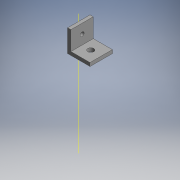
# Autodesk Inventor part: Part5
Saved by Autodesk Inventor 2016 (Build 200138000, 138)
## iProperties
Created: 2018-01-23
Part Number: Part5
Material: Generic
Document SubType Name: Modeling
Designer: student
Density: 1 g/cm^3
Appearance: Default
Author: student
Autodesk Inventor part; units mm, degrees
ref_plane "YZ Plane" through (0, 0, 0) normal (1, 0, 0) x (0, 1, 0)
ref_plane "XZ Plane" through (0, 0, 0) normal (0, 1, 0) x (-1, 0, 0)
ref_plane "XY Plane" through (0, 0, 0) normal (0, 0, 1) x (1, 0, 0)
sketch "Sketch1" plane through (0, 0, 0) normal (1, 0, 0) x (0, 1, 0)
  circle A0 centre (77.4226, -114.2734) radius 1.75 projected
  line L0 (66.4726, -104.7484) -> (66.4726, -123.7984) projected
  line L1 (66.4726, -104.7484) -> (85.5226, -104.7484) projected
  line L2 (85.5226, -123.7984) -> (85.5226, -104.7484) projected
  line L3 (66.4726, -123.7984) -> (85.5226, -123.7984) projected
  point P0 (0, 0)
extrude "Extrusion1" add sketch "Sketch1" along normal blind 2.794
sketch "Sketch3" plane through (2.794, 0, 0) normal (1, 0, 0) x (0, 0, -1)
  line L0 (104.7484, 66.4726) -> (123.7984, 66.4726) projected
  line L1 (104.7484, 85.5226) -> (104.7484, 66.4726) projected
  line L2 (104.7484, 66.4726) -> (104.7484, 69.3936)
  line L3 (104.7484, 66.4726) -> (107.6694, 66.4726) construction
  line L4 (123.7984, 66.4726) -> (123.7984, 85.5226) projected
  line L5 (123.7984, 66.4726) -> (123.7984, 69.3936)
  line L6 (123.7984, 66.4726) -> (126.7194, 66.4726) construction
  line L7 (123.7984, 69.3936) -> (104.7484, 69.3936)
  point P0 (0, 0)
  dimension "d2" = 2.921
  dimension "d3" = 90
  dimension "d4" = 2.921
  dimension "d5" = 90
  constraints: 10 end point, 2 collinear, 2 horizontal, 2 perpendicular
  measures "d2" distance of L0.start L2.end
  measures "d3" angle of L3 L2
  measures "d4" distance of L0.end L5.end
  measures "d5" angle of L6 L5
extrude "Extrusion2" add sketch "Sketch3" along normal blind 16.256
sketch "Sketch4" plane through (2.794, 69.3936, -104.7484) normal (0, 1, 0) x (1, 0, 0)
  line L0 (16.256, 19.05) -> (16.256, 0) construction
  line L1 (16.256, 0) -> (16.256, 19.05) construction
  line L2 (16.256, 9.525) -> (7.406, 9.525) construction
  circle A0 centre (7.406, 9.525) radius 2.5
  point P0 (-2.794, -104.7484)
  dimension "d8" = 8.85
  dimension "d9" = 5
  constraints: 2 end point, 1 centre point, 1 coincident, 1 horizontal, 1 midpoint
  measures "d8" distance of L2.start L2.end
  measures "d9" diameter of A0
extrude "Extrusion3" cut sketch "Sketch4" against normal blind 16.256
body "Solid1"
